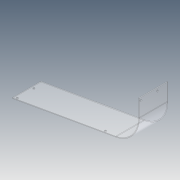
# Autodesk Inventor part: GE-12087-02
Saved by Autodesk Inventor 2012 (Build 160160000, 160)
## iProperties
Created: 2011-10-10
Part Number: GE-12087-02
Document SubType Name: Modeling
Designer: dfoster
Density: 1 g/cm^3
Description: Bottom
Material: Default
Title: Bottom
Author: dfoster
Autodesk Inventor part; units mm, degrees
ref_plane "YZ Plane" through (0, 0, 0) normal (1, 0, 0) x (0, 1, 0)
ref_plane "XZ Plane" through (0, 0, 0) normal (0, 1, 0) x (-1, 0, 0)
ref_plane "XY Plane" through (0, 0, 0) normal (0, 0, 1) x (1, 0, 0)
sketch "Sketch1" plane through (0, 0, 0) normal (0, 0, 1) x (1, 0, 0)
  line L0 (-325.0867, -79.7187) -> (100.1146, -4.7443) projected
  arc A0 (100.1146, -4.7443) -> (197.2008, 110.9585) centre (79.7131, 110.9585) ccw projected
  line L1 (197.2008, 110.9585) -> (197.2008, 182.1453) projected
  line L2 (194.0258, 182.1453) -> (197.2008, 182.1453) projected
  line L3 (194.0258, 182.1453) -> (194.0258, 110.9585) projected
  arc A1 (99.5632, -1.6175) -> (194.0258, 110.9585) centre (79.7131, 110.9585) ccw projected
  line L4 (99.5632, -1.6175) -> (-325.0867, -76.4948) projected
  line L5 (-325.0867, -79.7187) -> (-325.0867, -76.4948) projected
  point P0 (0, 0)
extrude "Extrusion1" add sketch "Sketch1" along normal blind 117.475
hole "Hole1" at (197.2008, 169.4453, 109.5375) direction (-1, 0, 0) diameter 6.731 depth 25.4 tip angle 118
pattern_linear "Rectangular Pattern1" count 2 spacing 68.2625 along (0, 0, -1) of "Hole1"
hole "Hole2" at (-312.5797, -77.5134, 109.5375) direction (-0.1736482, 0.9848078, 0) diameter 6.731 depth 25.4 tip angle 118
pattern_linear "Rectangular Pattern2" count 2 spacing 68.2625 along (0, 0, -1) of "Hole2"
pattern_linear "Rectangular Pattern3" count 2 spacing 368.3 along (0.9848078, 0.1736482, 0) of "Hole2"
body "Solid1"
